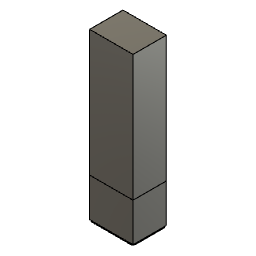
Tesying poles v6 (Autodesk Fusion 360 design; units mm, degrees)
Autodesk Fusion 360 part; units mm, degrees
sketch "Sketch1" plane through (0, 0, 0) normal (0, 1, 0) x (1, 0, 0)
  circle A0 centre (0, 0) radius 25
  circle A1 centre (0, 0) radius 28
  line L0 (40, -30) -> (-40, -30)
  line L1 (-40, -30) -> (-40, 30)
  line L2 (-40, 30) -> (40, 30)
  line L3 (40, 30) -> (40, -30)
  line L4 (40, -30) -> (-40, 30) construction
  line L5 (-40, -30) -> (40, 30) construction
  line L6 (43, -33) -> (-43, -33)
  line L7 (-43, -33) -> (-43, 33)
  line L8 (-43, 33) -> (43, 33)
  line L9 (43, 33) -> (43, -33)
  line L10 (43, -33) -> (-43, 33) construction
  line L11 (-43, -33) -> (43, 33) construction
  dimension "d1" = 50
  dimension "d2" = 56
  dimension "d3" = 80
  dimension "d4" = 60
  dimension "d5" = 86
  dimension "d6" = 66
  constraint coincident A0.centre A1.centre
  constraint concentric A0 A1
  constraint horizontal L0
  constraint perpendicular L0 L1
  constraint parallel L0 L2
  constraint parallel L1 L3
  constraint coincident L4 A0.centre
  constraint coincident L5 A0.centre
  constraint horizontal L6
  constraint perpendicular L6 L7
  constraint parallel L6 L8
  constraint parallel L7 L9
  constraint coincident L10 A0.centre
  constraint coincident L11 A0.centre
  measures "d1" diameter of A0
  measures "d2" diameter of A1
  measures "d3" distance of L1.end L2.end
  measures "d4" distance of L0.end L1.end
  measures "d5" distance of L7.end L8.end
  measures "d6" distance of L6.end L7.end
extrude "Extrude1" add sketch "Sketch1" along normal blind 250 contours L6 L7 L8 L9 makes body 1
sketch "Sketch2" plane through (0, 250, 0) normal (0, 1, 0) x (-1, 0, 0)
  line L0 (40, -30) -> (-40, -30)
  line L1 (-40, -30) -> (-40, 30)
  line L2 (-40, 30) -> (40, 30)
  line L3 (40, 30) -> (40, -30)
  line L4 (-43, -33) -> (43, -33)
  line L5 (43, -33) -> (43, 33)
  line L6 (43, 33) -> (-43, 33)
  line L7 (-43, 33) -> (-43, -33)
extrude "Extrude2" add sketch "Sketch2" against normal blind 3 contours L0 L1 L2 L3 | L4 L5 L6 L7 bodies 1
extrude "Extrude3" add sketch "Sketch1" along normal blind 250 separate body contours A1 makes body 2
sketch "Sketch3" plane through (0, 250, 0) normal (0, 1, 0) x (-1, 0, 0)
  circle A0 centre (0, 0) radius 25
  circle A1 centre (0, 0) radius 28
extrude "Extrude4" add sketch "Sketch3" against normal blind 3 contours A0 | A1 bodies 2
sketch "Sketch4" plane through (0, 0, 0) normal (0, -1, 0) x (1, 0, 0)
  circle A0 centre (0, 0) radius 25
  circle A1 centre (0, 0) radius 28
  circle A2 centre (0, 0) radius 12
  circle A3 centre (0, 0) radius 15
  dimension "d15" = 24
  dimension "d16" = 30
  constraint coincident A0.centre A1.centre
  constraint concentric A0 A3
  measures "d15" diameter of A2
  measures "d16" diameter of A3
extrude "Extrude5" add sketch "Sketch4" against normal blind 250 separate body contours A3 makes body 3
sketch "Sketch5" plane through (0, 250, 0) normal (0, 1, 0) x (-1, 0, 0)
  circle A0 centre (0, 0) radius 12
  circle A1 centre (0, 0) radius 15
extrude "Extrude6" add sketch "Sketch5" against normal blind 3 contours A0 bodies 3
move_body "Move1" bodies 1 to x (1, 0, 0) y (0, 1, 0) z (0, 0, 1) at (0, 6.4, 0)
move_body "Move2" bodies 2 to x (1, 0, 0) y (0, 1, 0) z (0, 0, 1) at (0, 3.2, 0)
sketch "Sketch6" plane through (0, 0, 0) normal (0, -1, 0) x (1, 0, 0)
  circle A0 centre (0, 0) radius 12
  circle A1 centre (0, 0) radius 15
  circle A2 centre (0, 0) radius 11.95
  circle A3 centre (0, 0) radius 25 construction
  line L0 (40, -30) -> (-40, -30) construction
  line L1 (-40, -30) -> (-40, 30) construction
  line L2 (-40, 30) -> (40, 30) construction
  line L3 (40, 30) -> (40, -30) construction
  line L4 (-43, -33) -> (43, -33) construction
  line L5 (43, -33) -> (43, 33) construction
  line L6 (43, 33) -> (-43, 33) construction
  line L7 (-43, 33) -> (-43, -33) construction
  circle A4 centre (0, 0) radius 24.9
  line L8 (39.9, 29.9) -> (39.9, -29.9)
  line L9 (39.9, -29.9) -> (-39.9, -29.9)
  line L10 (-39.9, -29.9) -> (-39.9, 29.9)
  line L11 (-39.9, 29.9) -> (39.9, 29.9)
  line L12 (-38.4, 28.4) -> (38.4, 28.4)
  line L13 (38.4, 28.4) -> (38.4, -28.4)
  line L14 (38.4, -28.4) -> (-38.4, -28.4)
  line L15 (-38.4, -28.4) -> (-38.4, 28.4)
  circle A5 centre (0, 0) radius 23
  circle A6 centre (0, 0) radius 10
  circle A7 centre (0, 0) radius 28
  line L16 (-43, -33) -> (43, -33)
  line L17 (-43, 33) -> (-43, -33)
  line L18 (43, 33) -> (-43, 33)
  line L19 (43, -33) -> (43, 33)
  dimension "d21" = -0.05
  dimension "d22" = -0.1
  dimension "d23" = 0.1
  dimension "d24" = 1.6
  dimension "d25" = -2
  dimension "d26" = -2
extrude "Extrude7" add sketch "Sketch6" along normal blind 70 separate body contours A0 | A1 | A2 makes body 4
extrude "Extrude8" add sketch "Sketch6" along normal blind 70 separate body contours A4 | L8 L9 L10 L11 | A7 | L16 L17 L18 L19 makes body 5 at (27.8609, -46.6667, -2.7879) makes body 6 at (-14.3333, -46.6667, -33)
extrude "Extrude9" add sketch "Sketch6" against normal blind 6.4 separate body contours L8 L9 L10 L11 | L16 L17 L18 L19 makes body 7
extrude "Extrude10" add sketch "Sketch6" against normal up to surface (3.2 mm away) separate body contours A4 | A7 makes body 8
combine "Combine1" operation add target body 6 tool bodies 7
combine "Combine2" operation add target body 5 tool bodies 8
extrude "Extrude11" add sketch "Sketch6" against normal blind 3 from surface at -6.4 contours L8 L9 L10 L11 bodies 6
extrude "Extrude12" add sketch "Sketch6" against normal blind 3 from surface at -3.2 contours A4 bodies 5
extrude "Extrude13" add sketch "Sketch6" against normal blind 3 contours A2 bodies 4
sketch "Sketch7" plane through (0, -70, 0) normal (0, -1, 0) x (1, 0, 0)
  line L0 (38.4, -28.4) -> (-38.4, -28.4)
  line L1 (-38.4, -28.4) -> (-38.4, 28.4)
  line L2 (-38.4, 28.4) -> (38.4, 28.4)
  line L3 (38.4, 28.4) -> (38.4, -28.4)
  line L4 (43, -33) -> (43, 33)
  line L5 (43, 33) -> (-43, 33)
  line L6 (-43, 33) -> (-43, -33)
  line L7 (-43, -33) -> (43, -33)
  line L8 (43, -33) -> (-43, -33)
  line L9 (-43, -33) -> (-43, 33)
  line L10 (-43, 33) -> (43, 33)
  line L11 (43, 33) -> (43, -33)
  line L12 (43, -33) -> (-43, 33) construction
  line L13 (-43, -33) -> (43, 33) construction
  circle A0 centre (0, 0) radius 23
  circle A1 centre (0, 0) radius 10
  constraint horizontal L8
  constraint perpendicular L8 L9
  constraint parallel L8 L10
  constraint parallel L9 L11
  constraint coincident L12 A0.centre
  constraint coincident L13 A0.centre
  constraint coincident L4.start L7.end
  constraint coincident A0.centre A1.centre
extrude "Extrude14" add sketch "Sketch7" along normal blind 2 contours L0 L1 L2 L3 | L4 L5 L6 L7 L8 L9 L10 L11 bodies 5
extrude "Extrude15" add sketch "Sketch7" along normal blind 2 contours L0 L1 L2 L3 | L4 L5 L6 L7 L8 L9 L10 L11 | A0 bodies 4
sketch "Sketch8" plane through (0, -70, 0) normal (0, -1, 0) x (1, 0, 0)
  line L0 (38.4, -28.4) -> (-38.4, -28.4)
  line L1 (-38.4, -28.4) -> (-38.4, 28.4)
  line L2 (-38.4, 28.4) -> (38.4, 28.4)
  line L3 (38.4, 28.4) -> (38.4, -28.4)
  line L4 (43, -33) -> (43, 33)
  line L5 (43, 33) -> (-43, 33)
  line L6 (-43, 33) -> (-43, -33)
  line L7 (-43, -33) -> (43, -33)
  circle A0 centre (0, 0) radius 28.4
  constraint coincident A0.centre origin
  constraint tangent L0 A0
extrude "Extrude16" add sketch "Sketch8" against normal blind 2 contours L0 L2 L3 A0 | L0 L1 L2 A0 bodies 6
fillet "Fillet1" radius 5 4 edges at (-43, -71, 33) (43, -71, 33) (-43, -71, -33) (43, -71, -33) on bodies 4
fillet "Fillet2" radius 5 4 edges at (-43, -71, -33) (-43, -71, 33) (43, -71, -33) (43, -71, 33) on bodies 5
sketch "Sketch9" plane through (0, 0, 0) normal (0, 1, 0) x (1, 0, 0)
  circle A0 centre (0, 0) radius 9
  circle A1 centre (0, 0) radius 6
  dimension "d53" = 18
  dimension "d54" = 12
  constraint coincident A0.centre A1.centre
  constraint concentric A0 A1
  measures "d53" diameter of A0
  measures "d54" diameter of A1
extrude "Extrude17" add sketch "Sketch9" along normal up to surface (246 mm away) separate body makes body 9
sketch "Sketch10" plane through (0, 246, 0) normal (0, 1, 0) x (-1, 0, 0)
  circle A0 centre (0, 0) radius 6
  circle A1 centre (0, 0) radius 9
extrude "Extrude18" add sketch "Sketch10" against normal blind 3 contours A0 bodies 9
sketch "Sketch11" plane through (0, 0, 0) normal (0, -1, 0) x (1, 0, 0)
  circle A0 centre (0, 0) radius 6
  circle A1 centre (0, 0) radius 9
  circle A2 centre (0, 0) radius 5.95
  circle A3 centre (0, 0) radius 4
  arc A4 (43, 28) -> (38, 33) centre (38, 28) ccw
  line L0 (38, 33) -> (-38, 33)
  arc A5 (-38, 33) -> (-43, 28) centre (-38, 28) ccw
  line L1 (-43, 28) -> (-43, -28)
  arc A6 (-43, -28) -> (-38, -33) centre (-38, -28) ccw
  line L2 (-38, -33) -> (38, -33)
  arc A7 (38, -33) -> (43, -28) centre (38, -28) ccw
  line L3 (43, -28) -> (43, 28)
  circle A8 centre (0, 0) radius 23
  dimension "d59" = -0.05
  dimension "d60" = -2
extrude "Extrude19" add sketch "Sketch11" against normal blind 10 separate body contours A2 makes body 10
extrude "Extrude20" add sketch "Sketch11" along normal up to surface (72 mm away) separate body contours A0 | A1 | A2 makes body 11
extrude "Extrude21" add sketch "Sketch11" against normal up to surface (2 mm away) from surface at 72 separate body contours A4 L0 A5 L1 A6 L2 A7 L3 | A8 makes body 12
combine "Combine3" operation add target body 12 tool bodies 11 10
named bodies: "Human", "Lightpole", "Lightpole_2", "Lightpole_2_bottom", "Lightpole_bottom", "Human_bottom", "Lightpole_3", "Lightpole_3_bottom"
